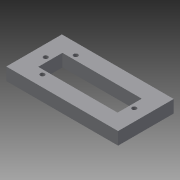
# Autodesk Inventor part: 490HV_SampleConnector
Saved by Autodesk Inventor 2015 (Build 190159000, 159)
## iProperties
Created: 2014-09-25
Part Number: 490HV_SampleConnector
Material: Generic
Document SubType Name: Modeling
Designer: Alex
Density: 1 g/cm^3
Appearance: Default
Author: Alex
Autodesk Inventor part; units mm, degrees
ref_plane "YZ Plane" through (0, 0, 0) normal (1, 0, 0) x (0, 1, 0)
ref_plane "XZ Plane" through (0, 0, 0) normal (0, 1, 0) x (-1, 0, 0)
ref_plane "XY Plane" through (0, 0, 0) normal (0, 0, 1) x (1, 0, 0)
sketch "Sketch1" plane through (0, 0, 0) normal (0, 1, 0) x (-1, 0, 0)
  line L0 (5.1091, 9.9192) -> (-42.0909, 9.9192)
  line L1 (-42.0909, 9.9192) -> (-42.0909, -13.5608)
  line L2 (-42.0909, -13.5608) -> (5.1091, -13.5608)
  line L3 (5.1091, -13.5608) -> (5.1091, 9.9192)
  point P0 (0, 0)
  dimension "d0" = 23.48
  dimension "d1" = 47.2
  constraints: 8 end point, 2 parallel, 1 horizontal, 1 perpendicular
  measures "d0" distance of L2.end L0.start
  measures "d1" distance of L1.end L2.end
extrude "Extrusion1" add sketch "Sketch1" along normal blind 5.31
sketch "Sketch2" plane through (0, 5.31, 0) normal (0, 1, 0) x (1, 0, 0)
  circle A0 centre (-0.1791, 1.8208) radius 0.93
  circle A1 centre (5.4509, -5.2092) radius 0.93
  line L0 (-5.1091, -9.9192) -> (42.0909, -9.9192) projected
  line L1 (42.0909, 13.5608) -> (-5.1091, 13.5608) projected
  circle A2 centre (5.4509, 8.8508) radius 0.93
  line L2 (-5.1091, 13.5608) -> (-5.1091, -9.9192) projected
  line L3 (42.0909, -9.9192) -> (42.0909, 13.5608) projected
  circle A3 centre (37.1609, 1.8208) radius 0.93
  point P0 (0, 0)
  dimension "d4" = 1.86
  dimension "d7" = 1.86
  dimension "d10" = 3.78
  dimension "d12" = 0
  dimension "d14" = 1.86
  dimension "d15" = 14.06
  dimension "d16" = 3.78
  dimension "d17" = 4
  dimension "d19" = 0
  dimension "d20" = 1.86
  dimension "d23" = 37.34
  dimension "d24" = 4
  dimension "d27" = 5.63
  dimension "d29" = 11.74
  dimension "d30" = 11.74
  constraints: 4 centre point
  measures "d4" diameter of A0
  measures "d7" diameter of A1
  measures "d10" distance edge to line of A1 L0
  measures "d12" horizontal distance of A2.centre A1.centre
  measures "d14" diameter of A2
  measures "d15" distance of A2.centre A1.centre
  measures "d16" distance edge to line of A2 L1
  measures "d17" distance edge to line of A0 L2
  measures "d19" vertical distance of A3.centre A0.centre
  measures "d20" diameter of A3
  measures "d23" distance of A0.centre A3.centre
  measures "d24" distance edge to line of A3 L3
  measures "d27" horizontal distance of A1.centre A0.centre
  measures "d29" distance from line of A0.centre L1
  measures "d30" distance from line of A3.centre L0
extrude "Extrusion2" cut sketch "Sketch2" against normal through all contours A0 | A1 | A2 | A3
sketch "Sketch3" plane through (0, 5.31, 0) normal (0, 1, 0) x (1, 0, 0)
  line L0 (1.7509, -3.2792) -> (35.2309, -3.2792)
  line L1 (35.2309, -3.2792) -> (35.2309, 6.9208)
  line L2 (35.2309, 6.9208) -> (1.7509, 6.9208)
  line L3 (1.7509, 6.9208) -> (1.7509, -3.2792)
  circle A0 centre (-0.1791, 1.8208) radius 0.93 projected
  circle A1 centre (5.4509, 8.8508) radius 0.93 projected
  circle A2 centre (5.4509, -5.2092) radius 0.93 projected
  circle A3 centre (37.1609, 1.8208) radius 0.93 projected
  point P0 (0, 0)
  dimension "d33" = 1
  dimension "d34" = 1
  dimension "d35" = 1
  dimension "d36" = 1
  constraints: 8 end point, 2 parallel, 1 horizontal, 1 perpendicular
  measures "d33" distance edge to line of A0 L3
  measures "d34" distance edge to line of A1 L2
  measures "d35" distance edge to line of A2 L0
  measures "d36" distance edge to line of A3 L1
extrude "Extrusion3" cut sketch "Sketch3" against normal through all contours L3 L2 L1 L0
body "Solid1"
